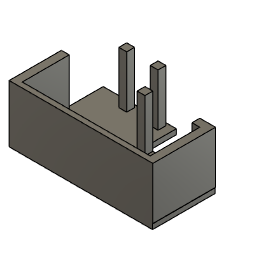
MountTest2 v1 (Autodesk Fusion 360 design; units mm, degrees)
Autodesk Fusion 360 part; units mm, degrees
sketch "草图1" plane through (0, 0, 0) normal (0, 1, 0) x (1, 0, 0)
  line L0 (0, 0) -> (6, 0)
  line L1 (6, 0) -> (6, 9.5)
  line L2 (0, 0) -> (-18.5, 0)
  line L3 (-18.5, 0) -> (-18.5, 9)
  line L4 (6, 9.5) -> (4.5, 9.5)
  line L5 (4.5, 9.5) -> (4.5, 11)
  line L6 (4.5, 11) -> (6, 11)
  line L7 (6, 11) -> (7.5, 11)
  line L8 (7.5, 11) -> (7.5, -1)
  line L9 (7.5, -1) -> (-20, -1)
  line L10 (-20, -1) -> (-20, 9)
  line L11 (-20, 9) -> (-18.5, 9)
  line L12 (-6, 11) -> (-6, 9.5)
  line L13 (-6, 9.5) -> (-4.5, 9.5)
  line L14 (-4.5, 9.5) -> (-4.5, 11)
  line L15 (-4.5, 11) -> (-6, 11)
  line L16 (-13.5, 15) -> (-15, 15)
  line L17 (-15, 15) -> (-15, 16.5)
  line L18 (-15, 16.5) -> (-13.5, 16.5)
  line L19 (-13.5, 16.5) -> (-13.5, 15)
  line L20 (-9, 16.5) -> (-7.5, 16.5)
  line L21 (-7.5, 16.5) -> (-7.5, 15)
  line L22 (-7.5, 15) -> (-9, 15)
  line L23 (-9, 15) -> (-9, 16.5)
  dimension "d1" = 6
  dimension "d2" = 9.5
  dimension "d3" = 18.5
  dimension "d4" = 9
  constraint coincident L0.start L2.start
  constraint horizontal L0
  constraint perpendicular L0 L1
  constraint parallel L0 L2
  constraint perpendicular L2 L3
  constraint perpendicular L1 L4
  constraint perpendicular L4 L5
  constraint perpendicular L5 L6
  constraint perpendicular L5 L7
  constraint perpendicular L7 L8
  constraint perpendicular L8 L9
  constraint perpendicular L9 L10
  constraint perpendicular L10 L11
  constraint perpendicular L4 L12
  constraint perpendicular L12 L13
  constraint perpendicular L4 L14
  constraint perpendicular L12 L15
  constraint horizontal L16
  constraint vertical L17
  constraint horizontal L18
  constraint vertical L19
  constraint horizontal L20
  constraint vertical L21
  constraint horizontal L22
  constraint vertical L23
  measures "d1" distance of L0.start L0.end
  measures "d2" distance of L0.end L1.end
  measures "d3" distance of L0.start L2.end
  measures "d4" distance of L2.end L3.end
sketch "草图2" plane through (0, 0, 0) normal (0, 1, 0) x (1, 0, 0)
  line L0 (-20, -1) -> (-20, 17)
  line L1 (-20, 17) -> (-6, 17)
  line L2 (-6, 17) -> (-6, 11)
  line L3 (-6, 11) -> (7.4403, 11)
  line L4 (7.4403, 11) -> (7.4403, -1)
  line L5 (7.4403, -1) -> (-20, -1)
  constraint vertical L0
  constraint perpendicular L0 L1
  constraint perpendicular L1 L2
  constraint perpendicular L2 L3
  constraint perpendicular L3 L4
  constraint perpendicular L0 L5
extrude "拉伸1" add sketch "草图2" against normal blind 1
extrude "拉伸2" add sketch "草图1" along normal blind 10
